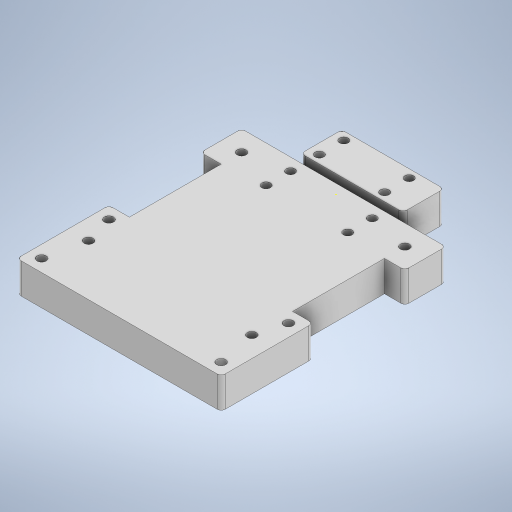
# Autodesk Inventor part: DerzavkaDviz
Saved by Autodesk Inventor 2024 (Build 280153000, 153)
## iProperties
Created: 2023-11-07
Part Number: DerzavkaDviz
Material: Generic
Document SubType Name: Modeling
Designer: KirikDK
Density: 1 g/cm^3
Appearance: Default
Author: KirikDK
Autodesk Inventor part; units mm, degrees
ref_plane "YZ Plane" through (0, 0, 0) normal (1, 0, 0) x (0, 1, 0)
ref_plane "XZ Plane" through (0, 0, 0) normal (0, 1, 0) x (-1, 0, 0)
ref_plane "XY Plane" through (0, 0, 0) normal (0, 0, 1) x (1, 0, 0)
sketch "Sketch1" plane through (0, 0, 0) normal (0, 1, 0) x (-1, 0, 0)
  line L0 (51.1111, 105.2222) -> (-48.8889, 105.2222)
  line L1 (-48.8889, 105.2222) -> (-48.8889, -4.7778)
  line L2 (-48.8889, -4.7778) -> (51.1111, -4.7778)
  line L3 (51.1111, -4.7778) -> (51.1111, 105.2222)
  line L4 (52.6672, 60.2222) -> (41.1111, 60.2222)
  line L5 (41.1111, 60.2222) -> (41.1111, 15.2222)
  line L6 (41.1111, 15.2222) -> (52.6672, 15.2222)
  line L7 (52.6672, 15.2222) -> (52.6672, 60.2222)
  line L8 (-66.472, 60.2222) -> (-38.8889, 60.2222)
  line L9 (-38.8889, 60.2222) -> (-38.8889, 15.2222)
  line L10 (-38.8889, 15.2222) -> (-66.472, 15.2222)
  line L11 (-66.472, 15.2222) -> (-66.472, 60.2222)
  point P0 (0, 0)
  point P1 (-48.8889, 60.2222)
  point P2 (-48.8889, 15.2222)
  point P3 (51.1111, 15.2222)
  point P4 (51.1111, 60.2222)
  dimension "d0" = 100
  dimension "d1" = 110
  dimension "d6" = 20
  dimension "d7" = 20
  dimension "d8" = 10
  dimension "d9" = 10
  dimension "d10" = 45
  dimension "d11" = 45
  constraints: 24 end point, 6 parallel, 3 horizontal, 3 perpendicular
  measures "d0" distance of L0.start L0.end
  measures "d1" distance of L2.end L0.start
  measures "d6" distance between parallel lines of L2 L10
  measures "d7" distance between parallel lines of L2 L6
  measures "d8" distance between parallel lines of L3 L5
  measures "d9" distance between parallel lines of L1 L9
  measures "d10" distance of L8.end L9.end
  measures "d11" distance of L4.end L5.end
extrude "Extrusion1" add sketch "Sketch1" along normal blind 15 contours L3 L4 L5 L6 L2 L1 L10 L9 L8 L0
sketch "Sketch2" plane through (0, 15, 0) normal (0, 1, 0) x (1, 0, 0)
  point P0 (0, 0)
sketch "Sketch3" plane through (0, 15, 0) normal (0, 1, 0) x (1, 0, 0)
  point P0 (0, 0)
sketch "Sketch4" plane through (0, 15, 0) normal (0, 1, 0) x (1, 0, 0)
  line L0 (48.8889, -105.2222) -> (48.8889, -60.2222) projected
  line L1 (48.8889, -60.2222) -> (38.8889, -60.2222) projected
  line L2 (38.8889, -60.2222) -> (38.8889, -15.2222) projected
  line L3 (38.8889, -15.2222) -> (48.8889, -15.2222) projected
  line L4 (48.8889, -15.2222) -> (48.8889, 4.7778) projected
  line L5 (48.8889, 4.7778) -> (-51.1111, 4.7778) projected
  line L6 (-51.1111, 4.7778) -> (-51.1111, -15.2222) projected
  line L7 (-51.1111, -15.2222) -> (-41.1111, -15.2222) projected
  line L8 (-41.1111, -15.2222) -> (-41.1111, -60.2222) projected
  line L9 (-41.1111, -60.2222) -> (-51.1111, -60.2222) projected
  line L10 (-51.1111, -60.2222) -> (-51.1111, -105.2222) projected
  line L11 (-51.1111, -105.2222) -> (48.8889, -105.2222) projected
  circle A0 centre (-41.1111, -5.2222) radius 10
  circle A1 centre (38.8889, -5.2222) radius 10
  circle A2 centre (-41.1111, -80.2222) radius 10
  circle A3 centre (38.8889, -80.2222) radius 10
  circle A4 centre (-41.1111, -80.2222) radius 2.1886
  circle A5 centre (38.8889, -80.2222) radius 2.1886
  circle A6 centre (-41.1111, -5.2222) radius 2.1886
  circle A7 centre (38.8889, -5.2222) radius 2.1886
  circle A8 centre (-21.1111, -13.2222) radius 2.1
  circle A9 centre (18.8889, -13.2222) radius 2.1
  line L12 (-45.1111, -99.2222) -> (-45.1111, -66.2222)
  line L13 (-45.1111, -66.2222) -> (-35.1111, -66.2222)
  line L14 (-35.1111, -66.2222) -> (-35.1111, -9.2222)
  line L15 (-35.1111, -9.2222) -> (-45.1111, -9.2222)
  line L16 (-45.1111, -9.2222) -> (-45.1111, -1.2222)
  line L17 (-45.1111, -1.2222) -> (42.8889, -1.2222)
  line L18 (42.8889, -1.2222) -> (42.8889, -9.2222)
  line L19 (42.8889, -9.2222) -> (32.8889, -9.2222)
  line L20 (32.8889, -9.2222) -> (32.8889, -66.2222)
  line L21 (32.8889, -66.2222) -> (42.8889, -66.2222)
  line L22 (42.8889, -66.2222) -> (42.8889, -99.2222)
  line L23 (42.8889, -99.2222) -> (-45.1111, -99.2222)
  circle A10 centre (-45.1111, -66.2222) radius 2.2222
  circle A11 centre (42.8889, -66.2222) radius 2.2222
  circle A12 centre (42.8889, -99.2222) radius 2.2222
  circle A13 centre (-45.1111, -99.2222) radius 2.2222
  circle A14 centre (-21.1111, -1.2222) radius 2.1
  circle A15 centre (18.8889, -1.2222) radius 2.1
  point P0 (0, 0)
  dimension "d19" = 20
  dimension "d20" = 20
  dimension "d21" = 10
  dimension "d22" = 10
  dimension "d23" = 18
  dimension "d24" = 18
  dimension "d25" = 20
  dimension "d26" = 20
  dimension "d27" = 4.2
  dimension "d28" = 4.2
  dimension "d29" = 6
  dimension "d38" = 12
  dimension "d39" = 12
  constraints: 24 end point, 16 centre point, 8 coincident, 8 tangent, 11 other
  measures "d19" distance from line of L9 A2.centre
  measures "d20" distance from line of L1 A3.centre
  measures "d21" distance from line of L0 A3.centre
  measures "d22" distance from line of L10 A2.centre
  measures "d23" distance from line of L5 A8.centre
  measures "d24" distance from line of L5 A9.centre
  measures "d25" distance from line of L8 A8.centre
  measures "d26" distance from line of L2 A9.centre
  measures "d27" diameter of A8
  measures "d28" diameter of A9
  measures "d29" distance between parallel lines of L10 L12
  measures "d38" distance of A14.centre A8.centre
  measures "d39" distance of A15.centre A9.centre
extrude "Extrusion2" cut sketch "Sketch4" against normal blind 15 contours A11 L21 L22 | L22 L21 A11 | A12 L23 L22 | L22 L23 A12 | A10 L13 L12 | L12 L13 A10 | A13 L23 L12 | L12 L23 A13 | A15 L17 | L17 A15 | A14 L17 | L17 A14 | A4 | A5 | A6 | A7 | A8 | A9
sketch "Sketch6" plane through (0, 15, 0) normal (0, 1, 0) x (1, 0, 0)
  line L0 (-26.1111, 8.8778) -> (23.8889, 8.8778)
  line L1 (23.8889, 8.8778) -> (23.8889, 28.8778)
  line L2 (23.8889, 28.8778) -> (-26.1111, 28.8778)
  line L3 (-26.1111, 28.8778) -> (-26.1111, 8.8778)
  line L4 (-51.1111, 4.7778) -> (-51.1111, -15.2222) projected
  line L5 (48.8889, -15.2222) -> (48.8889, 4.7778) projected
  line L6 (48.8889, 4.7778) -> (-51.1111, 4.7778) projected
  circle A0 centre (-21.1111, 24.8778) radius 2.1
  circle A1 centre (10.8889, 24.8778) radius 2.1
  circle A2 centre (-21.1111, 12.8778) radius 2.1
  circle A3 centre (10.8889, 12.8778) radius 2.1
  point P0 (0, 0)
  point P1 (-51.1111, -5.2222)
  dimension "d30" = 25
  dimension "d31" = 25
  dimension "d32" = 4.1
  dimension "d33" = 20
  dimension "d34" = 4
  dimension "d35" = 4
  dimension "d36" = 4
  dimension "d37" = 4
  constraints: 8 end point, 4 centre point, 2 parallel, 1 horizontal, 1 midpoint, 1 perpendicular
  measures "d30" distance from line of point (-51.111, -5.222) L3
  measures "d31" distance between parallel lines of L5 L1
  measures "d32" distance between parallel lines of L6 L0
  measures "d33" distance between parallel lines of L0 L2
  measures "d34" distance from line of L2 A0.centre
  measures "d35" distance from line of L2 A1.centre
  measures "d36" distance from line of L0 A3.centre
  measures "d37" distance from line of L0 A2.centre
extrude "Extrusion4" add sketch "Sketch6" against normal blind 15
fillet "Fillet1" radius 2 12 edges at (48.8889, 7.5, 60.2222) (48.8889, 7.5, 15.2222) (23.8889, 7.5, -8.8778) (23.8889, 7.5, -28.8778) (-26.1111, 7.5, -28.8778) (-26.1111, 7.5, -8.8778) (-51.1111, 7.5, -4.7778) (-51.1111, 7.5, 15.2222) (-51.1111, 7.5, 60.2222) (-51.1111, 7.5, 105.2222) (48.8889, 7.5, 105.2222) (48.8889, 7.5, -4.7778)
body "Solid1"
